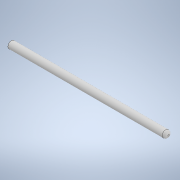
# Autodesk Inventor part: LightsaberBasicBladeButBad
Saved by Autodesk Inventor 2021 (Build 250183000, 183)
## iProperties
Created: 2021-03-22
Part Number: LightsaberBasicBladeButBad
Material: Générique
Document SubType Name: Modeling
Designer: turnb
Density: 1 g/cm^3
Appearance: Par défaut
Author: turnb
Autodesk Inventor part; units mm, degrees
ref_plane "YZ Plane" through (0, 0, 0) normal (1, 0, 0) x (0, 1, 0)
ref_plane "XZ Plane" through (0, 0, 0) normal (0, 1, 0) x (-1, 0, 0)
ref_plane "XY Plane" through (0, 0, 0) normal (0, 0, 1) x (1, 0, 0)
sketch "Esquisse1" plane through (0, 0, 0) normal (0, 0, 1) x (1, 0, 0)
  line L0 (0, 0) -> (540, 0)
  line L1 (550, 10) -> (550, 15)
  line L2 (540, 25) -> (0, 25)
  line L3 (0, 25) -> (0, 0)
  arc A0 (550, 15) -> (540, 25) centre (540, 15) ccw
  arc A1 (540, 0) -> (550, 10) centre (540, 10) ccw
  line L4 (0, 12.5) -> (550, 12.5)
  point P0 (550, 25)
  point P1 (550, 0)
  dimension "d0" = 550
  dimension "d1" = 25
  dimension "d2" = 10
  constraints: 10 end point, 4 point on circle, 4 point on line, 4 tangent, 2 centre point, 2 midpoint, 2 parallel, 1 equal radius, 1 horizontal, 1 perpendicular
  measures "d0" distance of L2.end point (550, 25)
  measures "d1" distance of point (550, 0) point (550, 25)
  measures "d2" radius of A0
revolve "Révolution1" add sketch "Esquisse1" angle 360 about axis through (0, 12.5, 0) along (1, 0, 0) contours L3 L2 A0 L1 L4
